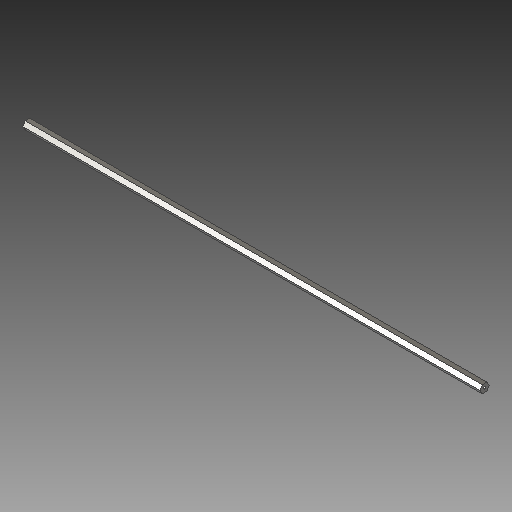
# Autodesk Inventor part: driveshaft
Saved by Autodesk Inventor 2017 SP1 (Build 210196100, 196)
## iProperties
Created: 2018-01-30
Part Number: driveshaft
Material: Steel
Document SubType Name: Modeling
Designer: Ben
Density: 7.85 g/cm^3
Appearance: Chrome - Polished
Mass: 318.766 g
Surface Area: 227.838 cm^2
Volume: 40.6071 cm^3
Author: Ben
Autodesk Inventor part; units mm, degrees
ref_plane "YZ Plane" through (0, 0, 0) normal (1, 0, 0) x (0, 1, 0)
ref_plane "XZ Plane" through (0, 0, 0) normal (0, 1, 0) x (-1, 0, 0)
ref_plane "XY Plane" through (0, 0, 0) normal (0, 0, 1) x (1, 0, 0)
sketch "Sketch1" plane through (0, 0, 0) normal (1, 0, 0) x (0, 1, 0)
  line L0 (0, -5.4993) -> (-4.7625, -2.7496)
  line L1 (-4.7625, -2.7496) -> (-4.7625, 2.7496)
  line L2 (-4.7625, 2.7496) -> (0, 5.4993)
  line L3 (0, 5.4993) -> (4.7625, 2.7496)
  line L4 (4.7625, 2.7496) -> (4.7625, -2.7496)
  line L5 (4.7625, -2.7496) -> (0, -5.4993)
  circle A0 centre (0, 0) radius 1.27
  dimension "d3" = 9.525
  dimension "d4" = 2.54
  constraints: 12 end point, 2 coincident, 1 centre point, 1 vertical, 13 other
  measures "d3" distance between parallel lines of L1 L4
  measures "d4" diameter of A0
extrude "Extrusion1" add sketch "Sketch1" along normal mid plane 552.45
body "Solid1"
